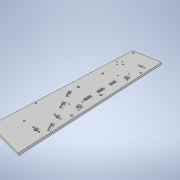
# Autodesk Inventor part: ChassisOutide10
Saved by Autodesk Inventor 2020 (Build 240168000, 168)
## iProperties
Created: 2019-10-11
Part Number: ChassisOutide10
Material: Generic
Document SubType Name: Modeling
Designer: shrey
Density: 1 g/cm^3
Appearance: Default
Author: shrey
Autodesk Inventor part; units mm, degrees
ref_plane "YZ Plane" through (0, 0, 0) normal (1, 0, 0) x (0, 1, 0)
ref_plane "XZ Plane" through (0, 0, 0) normal (0, 1, 0) x (-1, 0, 0)
ref_plane "XY Plane" through (0, 0, 0) normal (0, 0, 1) x (1, 0, 0)
sketch "Sketch1" plane through (0, 0, 0) normal (0, 1, 0) x (-1, 0, 0)
  line L0 (44.45, 203.2) -> (-44.45, 203.2)
  line L1 (-44.45, 203.2) -> (-44.45, -203.2)
  line L2 (-44.45, -203.2) -> (44.45, -203.2)
  line L3 (44.45, -203.2) -> (44.45, 203.2)
  line L4 (44.45, 203.2) -> (-44.45, -203.2) construction
  line L5 (-44.45, 203.2) -> (-20.955, 203.2)
  line L6 (-20.955, 203.2) -> (-20.955, 88.9) construction
  line L7 (-44.45, 88.9) -> (-44.45, 203.2)
  line L8 (44.45, 203.2) -> (44.45, 111.6492)
  line L9 (44.45, 203.2) -> (44.45, 38.1)
  line L10 (44.45, 38.1) -> (22.225, 38.1) construction
  line L11 (0, 203.2) -> (-66.675, 203.2)
  line L12 (-66.675, 203.2) -> (-66.675, 88.9) construction
  line L13 (-66.675, 203.2) -> (-66.675, 209.55) construction
  line L14 (-20.955, 114.3) -> (-20.955, 152.4) construction
  circle A0 centre (-20.955, 152.4) radius 8.001 construction
  circle A1 centre (-20.955, 152.4) radius 4.0005
  circle A2 centre (-20.955, 160.401) radius 1.85
  line L15 (17.145, 152.4) -> (-20.955, 152.4) construction
  circle A3 centre (-28.956, 152.4) radius 1.85
  line L16 (-20.955, 190.5) -> (-20.955, 152.4) construction
  circle A4 centre (-20.955, 144.399) radius 1.85
  line L17 (-59.055, 152.4) -> (-20.955, 152.4) construction
  circle A5 centre (-12.954, 152.4) radius 1.85
  line L18 (44.45, 0) -> (-44.45, 0) construction
  circle A6 centre (22.225, -63.5) radius 2.9766
  line L19 (32.5679, 18.912) -> (22.7595, 35.2429) construction
  line L20 (22.7595, 35.2429) -> (17.8553, 43.4083) construction
  line L21 (15.6729, 53.2085) -> (25.4813, 36.8776)
  line L22 (25.4813, 36.8776) -> (20.0377, 33.6081)
  line L23 (20.0377, 33.6081) -> (10.2292, 49.939)
  line L24 (10.2292, 49.939) -> (15.6729, 53.2085)
  line L25 (15.6729, 53.2085) -> (20.0377, 33.6081) construction
  line L26 (25.4813, 36.8776) -> (10.2292, 49.939) construction
  circle A7 centre (-20.955, -104.394) radius 1.5
  circle A8 centre (-34.3732, -81.153) radius 1.5
  circle A9 centre (-7.5368, -81.153) radius 1.5
  circle A10 centre (-28.067, -88.9) radius 5.9944
  circle A11 centre (-20.955, -152.4) radius 4.0005
  circle A12 centre (-28.956, -152.4) radius 1.85
  circle A13 centre (-12.954, -152.4) radius 1.85
  circle A14 centre (-37.0613, -128.2) radius 2.9766
  line L27 (-28.067, 88.9) -> (-44.45, 88.9) construction
  line L28 (-44.45, 88.9) -> (-44.45, 12.7)
  line L29 (44.45, 203.2) -> (34.925, 203.2)
  line L30 (34.925, 203.2) -> (34.925, 193.675) construction
  line L31 (34.925, 193.675) -> (44.45, 193.675) construction
  line L32 (44.45, 193.675) -> (44.45, 203.2)
  circle A15 centre (34.925, 193.675) radius 3.175
  line L33 (-44.45, 0) -> (-31.75, 0)
  circle A16 centre (-31.75, 0) radius 3.175
  circle A17 centre (34.925, -193.675) radius 3.175
  line L34 (-44.45, 0) -> (-19.455, 0) construction
  line L35 (-16.28, -76.0639) -> (-22.63, -76.0639) construction
  line L36 (-22.63, -76.0639) -> (-22.63, 51.9267) construction
  line L37 (-22.63, 51.9267) -> (-16.28, 51.9267) construction
  line L38 (-16.28, 51.9267) -> (-16.28, -76.0639) construction
  line L39 (-16.28, -2.5436) -> (-22.63, -2.5436)
  line L40 (-22.63, -2.5436) -> (-22.63, -21.5936)
  line L41 (-22.63, -21.5936) -> (-16.28, -21.5936)
  line L42 (-16.28, -21.5936) -> (-16.28, -2.5436)
  line L43 (-16.28, -40.6436) -> (-22.63, -40.6436)
  line L44 (-16.28, -59.6936) -> (-16.28, -40.6436)
  line L45 (-22.63, -40.6436) -> (-22.63, -59.6936)
  line L46 (-22.63, -59.6936) -> (-16.28, -59.6936)
  line L47 (-16.28, 35.5564) -> (-22.63, 35.5564)
  line L48 (-16.28, 16.5064) -> (-16.28, 35.5564)
  line L49 (-22.63, 35.5564) -> (-22.63, 16.5064)
  line L50 (-22.63, 16.5064) -> (-16.28, 16.5064)
  line L51 (-16.28, -2.5436) -> (-22.63, -2.5436)
  line L52 (-16.28, -21.5936) -> (-16.28, -2.5436)
  line L53 (-22.63, -2.5436) -> (-22.63, -21.5936)
  line L54 (-22.63, -21.5936) -> (-16.28, -21.5936)
  line L55 (44.45, -203.2) -> (25.4, -203.2)
  line L56 (25.4, -203.2) -> (25.4, -128.2) construction
  line L57 (25.4, -128.2) -> (44.45, -128.2) construction
  line L58 (44.45, -128.2) -> (44.45, -203.2)
  circle A18 centre (25.4, -128.2) radius 6.35 construction
  circle A19 centre (25.4, -128.2) radius 9.779 construction
  circle A20 centre (15.621, -128.2) radius 1.778
  circle A21 centre (25.4, -128.2) radius 6.35 construction
  circle A22 centre (25.4, -128.2) radius 9.779 construction
  line L59 (100.4, -128.2) -> (25.4, -128.2) construction
  line L60 (25.4, -128.2) -> (25.4, -109.15) construction
  circle A23 centre (25.4, -137.979) radius 1.778
  circle A24 centre (25.4, -128.2) radius 6.35 construction
  circle A25 centre (25.4, -128.2) radius 9.779 construction
  line L61 (25.4, -53.2) -> (25.4, -128.2) construction
  line L62 (25.4, -128.2) -> (6.35, -128.2) construction
  circle A26 centre (35.179, -128.2) radius 1.778
  circle A27 centre (25.4, -128.2) radius 6.35 construction
  circle A28 centre (25.4, -128.2) radius 9.779 construction
  line L63 (-49.6, -128.2) -> (25.4, -128.2) construction
  line L64 (25.4, -128.2) -> (25.4, -147.25) construction
  circle A29 centre (25.4, -118.421) radius 1.778
  line L65 (22.225, 12.7) -> (22.225, 38.1) construction
  line L66 (-66.675, 209.55) -> (-66.675, 184.15) construction
  circle A30 centre (22.225, 12.7) radius 2.9718
  circle A31 centre (22.225, 12.7) radius 12.065 construction
  line L67 (-20.955, 152.4) -> (-20.955, 104.775) construction
  circle A32 centre (-20.955, 104.775) radius 8.001 construction
  circle A33 centre (-20.955, 112.776) radius 1.8542
  circle A34 centre (-20.955, 104.775) radius 8.001 construction
  circle A35 centre (-28.956, 104.775) radius 1.8542
  circle A36 centre (-20.955, 104.775) radius 8.001 construction
  circle A37 centre (-20.955, 96.774) radius 1.8542
  circle A38 centre (-20.955, 104.775) radius 8.001 construction
  circle A39 centre (-12.954, 104.775) radius 1.8542
  circle A40 centre (-20.955, 152.4) radius 31.75 construction
  circle A41 centre (-20.955, 104.775) radius 15.875 construction
  line L68 (-20.955, 104.775) -> (-20.955, 57.15) construction
  arc A42 (-34.3732, -81.153) -> (-7.5368, -81.153) centre (-20.955, -88.9) ccw construction
  circle A43 centre (-28.067, 57.15) radius 5.9944
  circle A44 centre (-20.955, 41.656) radius 1.5
  circle A45 centre (-7.5368, 64.897) radius 1.5
  circle A46 centre (-34.3732, 64.897) radius 1.5
  arc A47 (-34.3732, 64.897) -> (-7.5368, 64.897) centre (-20.955, 57.15) ccw construction
  circle A48 centre (-20.955, 57.15) radius 31.75 construction
  circle A49 centre (-20.955, -88.9) radius 31.75 construction
  circle A50 centre (-20.955, -152.4) radius 31.75 construction
  line L69 (-3.944, 85.8702) -> (-36.606, 140.3261) construction
  line L70 (-36.606, 140.3261) -> (-26.8074, 123.9893)
  line L71 (-26.8074, 123.9893) -> (-32.253, 120.7231)
  line L72 (-32.253, 120.7231) -> (-42.0516, 137.0599)
  line L73 (-42.0516, 137.0599) -> (-36.606, 140.3261)
  line L74 (-3.944, 85.8702) -> (5.8645, 69.5394)
  line L75 (-9.3876, 82.6008) -> (-3.944, 85.8702)
  line L76 (0.4208, 66.2699) -> (-9.3876, 82.6008)
  line L77 (5.8645, 69.5394) -> (0.4208, 66.2699)
  line L78 (-23.5608, 118.532) -> (-13.7524, 102.2011)
  line L79 (-29.0044, 115.2625) -> (-23.5608, 118.532)
  line L80 (-19.196, 98.9316) -> (-29.0044, 115.2625)
  line L81 (-13.7524, 102.2011) -> (-19.196, 98.9316)
  line L82 (-34.647, 137.0599) -> (7.8217, 162.5369) construction
  line L83 (7.8217, 162.5369) -> (43.4289, 103.1818) construction
  line L84 (43.4289, 103.1818) -> (0.9602, 77.7048) construction
  circle A51 centre (39.6875, 109.4185) radius 1.85
  circle A52 centre (12.793, 154.25) radius 1.85
  circle A53 centre (-20.955, 104.775) radius 4.0005
  circle A54 centre (-37.0613, -128.2) radius 13.335 construction
  line L85 (-37.0613, -128.2) -> (-37.0613, -128.2) construction
  circle A55 centre (-37.0613, 84.5115) radius 2.9766
  circle A56 centre (-37.0613, 84.5115) radius 13.335 construction
  point P0 (0, 0)
  point P1 (-19.455, -12.0686)
  point P2 (-34.2357, -82.6467)
  point P3 (-35.8454, -80.8658)
  dimension "d19" = 16.002
  dimension "d74" = 19.558
  dimension "d112" = 16.002
  dimension "d0" = 88.9
  dimension "d1" = 406.4
  dimension "d5" = 165.1
  dimension "d10" = 6.35
  dimension "d18" = 38.1
  dimension "d20" = 8.001
  dimension "d21" = 3.7
  dimension "d24" = 360
  dimension "d33" = 9.525
  dimension "d34" = 6.35
  dimension "d50" = 9.525
  dimension "d51" = 9.525
  dimension "d52" = 6.35
  dimension "d53" = 12.7
  dimension "d54" = 6.35
  dimension "d57" = 6.35
  dimension "d58" = 127.9906
  dimension "d59" = 6.35
  dimension "d60" = 19.05
  dimension "d63" = 38.1
  dimension "d66" = 38.1
  dimension "d71" = 75
  dimension "d72" = 19.05
  dimension "d73" = 12.7
  dimension "d75" = 3.556
  dimension "d78" = 360
  dimension "d84" = 25.4
  dimension "d85" = 5.9436
  dimension "d86" = 24.13
  dimension "d87" = 19.05
  dimension "d110" = 47.625
  dimension "d113" = 3.7084
  dimension "d116" = 360
  dimension "d118" = 63.5
  dimension "d119" = 31.75
  dimension "d120" = 47.625
  dimension "d135" = 63.5
  dimension "d136" = 63.5
  dimension "d137" = 63.5
  dimension "d138" = 63.5
  dimension "d139" = 19.05
  dimension "d140" = 6.35
  dimension "d143" = 38.1
  dimension "d150" = 3.7
  dimension "d151" = 3.7
  dimension "d154" = 8.001
  dimension "d157" = 26.67
  dimension "d178" = 26.67
  constraints: 172 end point, 48 centre point, 26 coincident, 17 parallel, 16 point on line, 10 perpendicular, 8 horizontal, 7 midpoint, 6 point on circle, 5 vertical alignment, 4 horizontal alignment, 4 symmetric about line, 3 vertical, 1 collinear, 141 other
  measures "d0" distance of L1.end L2.end
  measures "d1" distance of L0.end L1.end
  measures "d5" distance of L0.start L9.end
  measures "d10" distance of L11.end L13.end
  measures "d18" distance of L14.start L14.end
  measures "d20" diameter of A1
  measures "d21" diameter of A2
  measures "d33" distance of L20.start L20.end
  measures "d34" distance of L21.end L22.end
  measures "d50" distance of L30.end L31.end
  measures "d51" distance of L29.end L30.end
  measures "d52" diameter of A15
  measures "d53" distance of L18.end L33.end
  measures "d54" diameter of A16
  measures "d57" distance of L36.end L37.end
  measures "d58" distance of L35.end L36.end
  measures "d59" distance of L41.end L40.end
  measures "d60" distance of L40.end L39.end
  measures "d63" distance of L39.start L43.start
  measures "d66" distance of L39.start L47.start
  measures "d71" distance of L55.end L56.end
  measures "d72" distance of L56.end L57.end
  measures "d73" diameter of A18
  measures "d75" diameter of A20
  measures "d84" distance of L13.end L66.end
  measures "d85" diameter of A30
  measures "d86" diameter of A31
  measures "d87" distance of L19.start L19.end
  measures "d110" distance of L17.end L67.end
  measures "d113" diameter of A33
  measures "d118" diameter of A40
  measures "d119" diameter of A41
  measures "d120" distance of L68.start L68.end
  measures "d135" diameter of A48
  measures "d136" diameter of A49
  measures "d137" diameter of A50
  measures "d138" distance of L69.start L69.end
  measures "d139" distance of L69.end L70.end
  measures "d140" distance of L70.end L71.end
  measures "d143" distance of L21.start L74.start
  measures "d150" diameter of A51
  measures "d151" diameter of A52
  measures "d154" diameter of A53
  measures "d157" diameter of A54
  measures "d178" diameter of A56
extrude "Extrusion13" add sketch "Sketch1" along normal blind 6.35 contours L3 L2 L1 L0 | A2 | A4 | A33 L78 | L78 A33 | A33 L78 L81 L80 A53 L79 | A37
body "Solid13"
